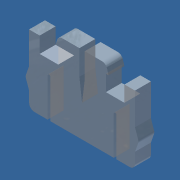
# Autodesk Inventor part: pressfit1press
Saved by Autodesk Inventor 2014 (Build 180170000, 170)
## iProperties
Created: 2013-09-11
Part Number: pressfit1press
Material: Glass
Document SubType Name: Modeling
Designer: Lefo
Density: 2.18 g/cm^3
Appearance: Clear
Author: Lefo
Autodesk Inventor part; units mm, degrees
ref_plane "YZ Plane" through (0, 0, 0) normal (1, 0, 0) x (0, 1, 0)
ref_plane "XZ Plane" through (0, 0, 0) normal (0, 1, 0) x (-1, 0, 0)
ref_plane "XY Plane" through (0, 0, 0) normal (0, 0, 1) x (1, 0, 0)
sketch "Sketch1" plane through (0, 0, 0) normal (0, 1, 0) x (-1, 0, 0)
  line L0 (0, 0) -> (20, 0)
  line L1 (20, 0) -> (20, 3)
  line L2 (20, 3) -> (0, 3)
  line L3 (0, 3) -> (0, 0)
  dimension "d0" = 20
  dimension "d1" = 3
  constraints: 8 end point, 2 parallel, 1 horizontal, 1 perpendicular
  measures "d0" distance of L2.end L1.end
  measures "d1" distance of L1.end L0.end
extrude "Extrusion1" add sketch "Sketch1" along normal blind 10
sketch "Sketch2" plane through (0, 10, 0) normal (0, 1, 0) x (1, 0, 0)
  line L0 (-20, 0) -> (-20, -3) projected
  line L1 (0, 0) -> (-20, 0) projected
  line L2 (-20, -3) -> (0, -3) projected
  line L3 (0, -3) -> (0, 0) projected
  line L4 (-14.5, 0) -> (-10.5, 0)
  line L5 (-10.5, 0) -> (-10.5, -3)
  line L6 (-10.5, -3) -> (-14.5, -3)
  line L7 (-14.5, -3) -> (-14.5, 0)
  line L8 (-9.5, 0) -> (-5.5, 0)
  line L9 (-5.5, 0) -> (-5.5, -3)
  line L10 (-5.5, -3) -> (-9.5, -3)
  line L11 (-9.5, -3) -> (-9.5, 0)
  line L12 (-10, 1.8071) -> (-10, -4.5751) construction
  dimension "d26" = 20
  dimension "d27" = 4
  dimension "d28" = 4
  dimension "d45" = 1
  dimension "d46" = 10
  dimension "d47" = 0.5
  constraints: 18 end point, 5 parallel, 4 point on line, 2 horizontal, 2 perpendicular
  measures "d26" distance of L1.start L0.start
  measures "d27" distance of L4.start L4.end
  measures "d28" distance of L9.end L10.end
  measures "d45" distance between parallel lines of L11 L5
  measures "d46" distance between parallel lines of L12 L0
  measures "d47" distance between parallel lines of L12 L5
extrude "Extrusion2" add sketch "Sketch2" along normal blind 3 contours L1 L5 L2 L7 | L1 L9 L2 L11
sketch "Sketch5" plane through (0, 0, 0) normal (0, 0, -1) x (-1, 0, 0)
  line L0 (0, 0) -> (20, 0) projected
  line L1 (9.5, 10) -> (10.5, 10) projected
  line L2 (16.2, 7.5) -> (16.3, 7.5)
  line L3 (16.5, 7.3) -> (16.5, 0)
  line L4 (16.5, 0) -> (16, 0)
  line L5 (16, 0) -> (16, 7.3)
  line L6 (10, 10) -> (10, 0) construction
  arc A0 (16.2, 7.5) -> (16, 7.3) centre (16.2, 7.3) ccw
  arc A1 (16.5, 7.3) -> (16.3, 7.5) centre (16.3, 7.3) ccw
  line L7 (3.8, 7.5) -> (3.7, 7.5)
  line L8 (3.5, 7.3) -> (3.5, 0)
  line L9 (3.5, 0) -> (4, 0)
  line L10 (4, 0) -> (4, 7.3)
  arc A2 (4, 7.3) -> (3.8, 7.5) centre (3.8, 7.3) ccw
  arc A3 (3.7, 7.5) -> (3.5, 7.3) centre (3.7, 7.3) ccw
  point P0 (16.5, 7.5)
  point P1 (3.5, 7.5)
  dimension "d61" = 0.5
  dimension "d62" = 7.5
  dimension "d63" = 6
  dimension "d64" = 0.2
  constraints: 18 end point, 9 symmetric about line, 8 point on circle, 4 centre point, 4 point on line, 4 tangent, 2 midpoint, 2 parallel, 1 collinear, 1 equal radius, 1 horizontal, 1 perpendicular, 2 other
  measures "d61" distance of L3.end L4.end
  measures "d62" distance of point (16.5, 7.5) L3.end
  measures "d63" distance between parallel lines of L5 L6
  measures "d64" radius of A0
extrude "Extrusion5" cut sketch "Sketch5" against normal blind 3
sketch "Sketch6" plane through (-20, 0, 0) normal (0, 0, -1) x (-1, 0, 0)
  line L0 (0, 0) -> (0, 10) projected
  line L1 (-5.5, 10) -> (0, 10) projected
  line L2 (-10.5, 10) -> (-9.5, 10) projected
  line L3 (-2.75, 10) -> (-2.75, 5) construction
  line L4 (-2.75, 5) -> (0, 5) construction
  line L5 (0, 5) -> (0.7, 5)
  line L6 (0, 5) -> (0, 7)
  line L7 (0, 7) -> (0.5844, 5.3304)
  line L8 (0, 5) -> (0, 3)
  line L9 (0, 3) -> (0.5844, 4.6696)
  arc A0 (0.5844, 4.6696) -> (0.5844, 5.3304) centre (-0.3595, 5) ccw
  line L10 (-16.5, 0) -> (-16.5, 7.3) projected
  line L11 (-16, 7.3) -> (-16, 0) projected
  line L12 (-10, 10) -> (-10, 0) construction
  line L13 (-20, 5) -> (-20, 7)
  line L14 (-20, 7) -> (-20.5844, 5.3304)
  line L15 (-20, 5) -> (-20, 3)
  line L16 (-20, 3) -> (-20.5844, 4.6696)
  arc A1 (-20.5844, 5.3304) -> (-20.5844, 4.6696) centre (-19.6405, 5) ccw
  dimension "d36" = 5
  dimension "d37" = 0.7
  dimension "d38" = 2
  dimension "d39" = 2
  dimension "d40" = 1
  constraints: 24 end point, 6 symmetric about line, 4 point on circle, 4 point on line, 3 midpoint, 2 centre point, 2 parallel, 2 tangent, 1 collinear, 1 other
  measures "d36" distance of L3.start L3.end
  measures "d37" distance of L4.end L5.end
  measures "d38" distance of L4.end L8.end
  measures "d39" distance of L4.end L6.end
  measures "d40" radius of A0
extrude "Extrusion6" add sketch "Sketch6" against normal blind 3
sketch "Sketch7" plane through (-5.5, 10, 3) normal (0, 0, 1) x (1, 0, 0)
  line L0 (-5, 0) -> (-4, 0) projected
  line L1 (-9, 3) -> (-5, 3) projected
  line L2 (-9, 0) -> (-9, 3) projected
  line L3 (-14.5, -10) -> (-11, -10) projected
  line L4 (-9, 3) -> (-9.5, 3)
  line L5 (-9.5, 3) -> (-9, 4.6927)
  line L6 (-9, 4.6927) -> (-5, 4.6927)
  line L7 (-5, 4.6927) -> (-5, 3)
  line L8 (-4.5, 0) -> (-4.5, 8.186) construction
  line L9 (0, 3) -> (-4, 3)
  line L10 (0, 3) -> (0.5, 3)
  line L11 (0.5, 3) -> (0, 4.6927)
  line L12 (0, 4.6927) -> (-4, 4.6927)
  line L13 (-4, 4.6927) -> (-4, 3)
  line L14 (-4.5, 0) -> (-4.5, -4) construction
  line L15 (-5, 0) -> (-4.5, -4)
  line L16 (-4, 0) -> (-4.5, -4)
  point P0 (-9, -10)
  dimension "d48" = 0.5
  dimension "d49" = 4
  constraints: 26 end point, 4 parallel, 3 symmetric about line, 1 midpoint, 1 perpendicular, 1 point on line
  measures "d48" distance of L1.start L4.end
  measures "d49" distance of L8.start L14.end
extrude "Extrusion7" add sketch "Sketch7" against normal blind 3 contours L4 L5 L6 L7 L1 | L9 L13 L12 L11 L10
extrude "Extrusion8" cut sketch "Sketch7" against normal blind 3 contours L0 L16 L15
fillet "Fillet1" radius 1 2 edges at (-5.5, 14.6927, 1.5) (-14.5, 14.6927, 1.5)
sketch "Sketch8" plane through (0, 10, 0) normal (0, 1, 0) x (1, 0, 0)
  line L0 (0, -3) -> (0, 0) projected
  line L1 (0, 0) -> (-5.5, 0) projected
  line L2 (-14.5, -3) -> (-14.5, 0) projected
  line L3 (-14.5, 0) -> (-20, 0) projected
  line L4 (-20, 0) -> (-20, -3) projected
  line L5 (-20, -3) -> (-14.5, -3) projected
  line L6 (-20, 0) -> (-18, 0)
  line L7 (-18, 0) -> (-18, -3)
  line L8 (-18, -3) -> (-20, -3)
  line L9 (-20, -3) -> (-20, 0)
  line L10 (-20, 0) -> (-20, -3) projected
  line L11 (-14.5, 0) -> (-20, 0) projected
  line L12 (-2, 0) -> (0, 0)
  line L13 (0, 0) -> (0, -3)
  line L14 (0, -3) -> (-2, -3)
  line L15 (-2, -3) -> (-2, 0)
  dimension "d55" = 2
  dimension "d56" = 3
  dimension "d57" = 2
  dimension "d58" = 3
  constraints: 16 end point, 4 collinear, 4 parallel, 2 horizontal, 2 perpendicular
  measures "d55" distance of L6.start L6.end
  measures "d56" distance of L6.end L7.end
  measures "d57" distance of L13.end L14.end
  measures "d58" distance of L12.end L13.end
extrude "Extrusion9" add sketch "Sketch8" along normal blind 3 contours L14 L15 L1 L0 | L5 L4 L3 L7
fillet "Fillet2" radius 1 2 edges at (0, 0, 1.5) (-20, 0, 1.5)
equation "\"d28\" = d27"
equation "\"d46\" = 0.5 * d26"
equation "\"d47\" = 0.5 * d45"
equation "\"d39\" = d38"
body "Solid1"
